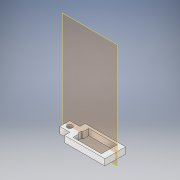
# Autodesk Inventor part: SG90 360 Degree Servo Holder
Saved by Autodesk Inventor 2019 (Build 230136000, 136)
## iProperties
Created: 2022-01-04
Part Number: SG90 360 Degree Servo Holder
Material: Generic
Description: STEP AP214
Document SubType Name: Modeling
Designer: Garrett Raker
Density: 1 g/cm^3
Appearance: Default
Sending System: SolidWorks 2020
Preprocessor: SwSTEP 2.0
Title: SG90 Servo.STEP
Revision Number: ANY
Autodesk Inventor part; units mm, degrees
ref_plane "YZ Plane" through (0, 0, 0) normal (1, 0, 0) x (0, 1, 0)
ref_plane "Work Plane1" through (-8.5267, 21.9678, 110.0832) normal (0, 0, 1) x (1, 0, 0)
sketch "Sketch1" plane through (-8.5267, 21.9678, 110.0832) normal (0, 0, 1) x (1, 0, 0)
  line L0 (3.95, 0) -> (3.95, -10.3) projected
  line L1 (3.95, 0) -> (3.95, -5.15)
  line L2 (4.8, 0) -> (4.8, -10.3) projected
  point P0 (8.5267, -21.9678)
  constraints: 2 end point, 1 parallel
ref_plane "Work Plane3" through (-8.5267, -54.2322, 21.6832) normal (0, -1, 0) x (1, 0, 0)
sketch "Sketch6" plane through (-8.5267, -54.2322, 21.6832) normal (0, -1, 0) x (1, 0, 0)
  line L0 (3.95, 0.85) -> (3.95, 11.35) projected
  line L1 (3.95, 12.3) -> (3.95, -0.1)
  line L2 (5.95, 4.6) -> (5.95, 7.6) projected
  line L3 (25.6, 12.1) -> (4.8, 12.1) construction
  line L4 (15.2, 12.1) -> (15.2, 0) construction
  line L5 (25.6, 0) -> (4.8, 0) construction
  line L6 (26.45, 12.3) -> (26.45, -0.1)
  line L7 (-0.85, 6.1) -> (31.25, 6.1) construction
  line L8 (31.25, 14.3) -> (-0.85, 14.3)
  line L9 (31.25, -2.1) -> (-0.85, -2.1)
  line L10 (-0.85, 14.3) -> (-0.85, -2.1)
  line L11 (31.25, 14.3) -> (31.25, -2.1)
  line L12 (3.95, 12.3) -> (26.45, 12.3)
  line L13 (3.95, -0.1) -> (26.45, -0.1)
  point P0 (5.95, 6.1)
  point P1 (3.95, 6.1)
  point P2 (-0.85, 6.1)
  point P3 (26.45, 6.1)
  point P4 (31.25, 6.1)
  dimension "d19" = 12.4
  constraints: 20 end point, 7 midpoint, 4 symmetric about line, 3 horizontal alignment, 2 vertical
  measures "d19" distance of L1.start L1.end
extrude "Extrusion4" add sketch "Sketch6" against normal blind 5
sketch "Sketch7" plane through (-8.5267, -54.2322, 21.6832) normal (0, -1, 0) x (1, 0, 0)
  line L0 (2.95, 4.6) -> (3.95, 4.6)
  line L1 (3.95, 4.6) -> (3.95, 7.6)
  line L2 (3.95, 7.6) -> (2.95, 7.6)
  line L3 (2.95, 7.6) -> (2.95, 4.6)
  line L4 (3.95, -0.1) -> (3.95, 12.3) projected
  line L5 (-0.85, 14.3) -> (-0.85, -2.1) projected
  point P0 (8.5267, -21.6832)
  point P1 (2.95, 6.1)
  point P2 (3.95, 6.1)
  dimension "d20" = 1
  dimension "d21" = 3
  constraints: 8 end point, 2 midpoint, 2 parallel, 1 collinear, 1 horizontal, 1 horizontal alignment, 1 perpendicular
  measures "d20" distance of L0.start L0.end
  measures "d21" distance between parallel lines of L2 L0
extrude "Extrusion5" cut sketch "Sketch7" against normal up to surface (5 mm away)
sketch "Sketch8" plane through (-8.5267, -54.2322, 21.6832) normal (0, -1, 0) x (1, 0, 0)
  line L0 (-0.85, 14.3) -> (-0.85, -2.1) projected
  line L1 (-0.85, 2.1) -> (-8.85, 2.1)
  line L2 (-8.85, 2.1) -> (-8.85, 10.1)
  line L3 (-8.85, 10.1) -> (-0.85, 10.1)
  line L4 (-0.85, 10.1) -> (-0.85, 2.1)
  line L5 (4.05, 11.35) -> (4.05, 0.85) projected
  circle A0 centre (-4.85, 6.1) radius 2
  point P0 (8.5267, -21.6832)
  point P1 (-8.85, 6.1)
  point P2 (4.05, 6.1)
  point P3 (-4.85, 2.1)
  dimension "d24" = 8
  dimension "d25" = 8
  dimension "d26" = 4
  constraints: 8 end point, 3 midpoint, 2 horizontal alignment, 2 parallel, 1 centre point, 1 horizontal, 1 perpendicular, 1 point on line, 1 vertical alignment
  measures "d24" distance of L1.end L2.end
  measures "d25" distance of L1.start L1.end
  measures "d26" diameter of A0
extrude "Extrusion6" add sketch "Sketch8" against normal up to surface (5 mm away)
ref_plane "Work Plane4" through (-4.5767, -54.2322, 27.7832) normal (0, 0, 1) x (1, 0, 0)
body "Solid1"
body "Solid14"
